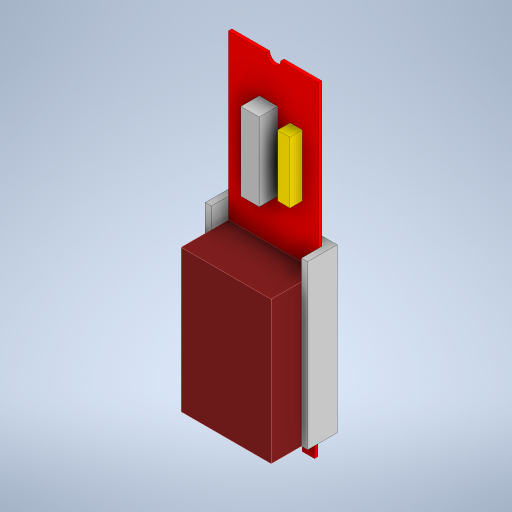
# Autodesk Inventor part: EGPL-T101-C1
Saved by Autodesk Inventor 2024.2 (Build 282272000, 272)
## iProperties
Created: 2024-02-23
Part Number: EGPL-T101-C1
Material: Generic
Document SubType Name: Modeling
Designer: lgnds
Density: 1 g/cm^3
Appearance: Default
Author: lgnds
Autodesk Inventor part; units mm, degrees
ref_plane "YZ Plane" through (0, 0, 0) normal (1, 0, 0) x (0, 1, 0)
ref_plane "XZ Plane" through (0, 0, 0) normal (0, 1, 0) x (-1, 0, 0)
ref_plane "XY Plane" through (0, 0, 0) normal (0, 0, 1) x (1, 0, 0)
sketch "Sketch1" plane through (0, 0, 0) normal (0, 0, 1) x (1, 0, 0)
  line L0 (-11, -40) -> (11, -40)
  line L1 (11, -40) -> (11, 40)
  line L2 (11, 40) -> (-11, 40)
  line L3 (-11, 40) -> (-11, -40)
  line L4 (-11, -40) -> (11, 40) construction
  line L5 (11, -40) -> (-11, 40) construction
  point P0 (0, 0)
  dimension "d0" = 22
  dimension "d1" = 80
  constraints: 12 end point, 2 midpoint, 2 parallel, 1 horizontal, 1 perpendicular
  measures "d0" distance of L1.end L2.end
  measures "d1" distance of L2.end L0.start
extrude "Extrusion1" add sketch "Sketch1" along normal blind 0.8
sketch "Sketch2" plane through (0, 0, 0.8) normal (0, 0, 1) x (1, 0, 0)
  line L0 (11, -40) -> (11, 40) projected
  line L1 (11, 40) -> (-11, 40) projected
  line L2 (-11, 40) -> (-11, -40) projected
  line L3 (-11, -40) -> (11, -40) projected
  line L4 (-10, -40) -> (-10, -36)
  line L5 (-10, -36) -> (-11, -36)
  line L6 (10, -40) -> (10, -36)
  line L7 (10, -36) -> (11, -36)
  line L8 (-7, -40) -> (-5, -40)
  line L9 (-5, -40) -> (-5, -36)
  line L10 (-5, -36) -> (-7, -36)
  line L11 (-7, -36) -> (-7, -40)
  line L12 (0, 56) -> (0, -56) construction
  line L13 (11, -40) -> (-11, -40)
  line L14 (7, -40) -> (5, -40)
  line L15 (5, -40) -> (5, -36)
  line L16 (5, -36) -> (7, -36)
  line L17 (7, -36) -> (7, -40)
  point P0 (0, 0)
  dimension "d4" = 1
  dimension "d5" = 1
  dimension "d6" = 4
  dimension "d7" = 2
  dimension "d8" = 3
  constraints: 26 end point, 9 point on line, 6 symmetric about line, 3 perpendicular, 2 parallel, 1 horizontal, 1 vertical
  measures "d4" distance between parallel lines of L2 L4
  measures "d5" distance between parallel lines of L0 L6
  measures "d6" distance between parallel lines of L3 L5
  measures "d7" distance between parallel lines of L11 L9
  measures "d8" distance between parallel lines of L4 L11
extrude "Extrusion2" cut sketch "Sketch2" against normal blind 0.8 contours L3 L6 L7 L0 | L3 L15 L16 L17 | L5 L4 L3 L2 | L3 L11 L10 L9
fillet "Fillet1" radius 1 5 edges at (-7, -36, 0.4) (-5, -36, 0.4) (5, -36, 0.4) (7, -36, 0.4) (10, -36, 0.4)
sketch "Sketch3" plane through (0, 0, 0.8) normal (0, 0, 1) x (1, 0, 0)
  line L0 (7, -37) -> (7, -40) projected
  line L1 (7, -40) -> (10, -40) projected
  line L2 (10, -40) -> (10, -37) projected
  arc A0 (11, -36) -> (10, -37) centre (11, -37) ccw projected
  line L3 (11, -36) -> (11, 40) projected
  line L4 (11, 40) -> (-11, 40) projected
  line L5 (-11, 40) -> (-11, -36) projected
  line L6 (-11, -36) -> (-10, -36) projected
  line L7 (-10, -36) -> (-10, -40) projected
  line L8 (-10, -40) -> (-7, -40) projected
  line L9 (-7, -40) -> (-7, -37) projected
  arc A1 (-5, -37) -> (-7, -37) centre (-6, -37) ccw projected
  line L10 (-5, -37) -> (-5, -40) projected
  line L11 (-5, -40) -> (5, -40) projected
  line L12 (5, -40) -> (5, -37) projected
  arc A2 (7, -37) -> (5, -37) centre (6, -37) ccw projected
  line L13 (11, -36) -> (11, 40) projected
  line L14 (-11, 0) -> (11, 0)
  line L15 (11, 0) -> (11, -34.8)
  line L16 (11, -34.8) -> (-11, -34.8)
  line L17 (-11, -34.8) -> (-11, 0)
  point P0 (0, 0)
  point P1 (11, 0)
  dimension "d12" = 5.2
  dimension "d13" = 40
  constraints: 8 end point, 2 parallel, 2 point on line, 1 horizontal, 1 perpendicular
  measures "d12" distance between parallel lines of L11 L16
  measures "d13" distance between parallel lines of L11 L14
extrude "Extrusion3" add sketch "Sketch3" along normal blind 11.6 separate body contours L16 L5 L14 L3
sketch "Sketch4" plane through (0, 0, 0) normal (0, 0, -1) x (-1, 0, 0)
  line L0 (-12.5, -34.8) -> (12.5, -34.8)
  line L1 (12.5, -34.8) -> (12.5, 5)
  line L2 (12.5, 5) -> (-12.5, 5)
  line L3 (-12.5, 5) -> (-12.5, -34.8)
  line L4 (11, -34.8) -> (-11, -34.8) projected
  line L5 (-11, -36) -> (-11, 40) projected
  line L6 (11, 40) -> (11, -36) projected
  line L7 (-7, -40) -> (-10, -40) projected
  point P0 (0, 0)
  point P1 (0, -34.8)
  point P2 (-8.5, -40)
  point P3 (11, 5)
  point P4 (-11, 5)
  dimension "d16" = 1.5
  dimension "d17" = 1.5
  dimension "d18" = 45
  constraints: 8 end point, 3 midpoint, 2 parallel, 1 horizontal, 1 perpendicular
  measures "d16" distance between parallel lines of L5 L3
  measures "d17" distance between parallel lines of L6 L1
  measures "d18" distance from line of point (-8.5, -40) L2
extrude "Extrusion4" add sketch "Sketch4" along normal blind 2.2 separate body
sketch "Sketch5" plane through (0, 0, 0) normal (0, 0, 1) x (1, 0, 0)
  line L0 (-12.5, 5) -> (12.5, 5) projected
  line L1 (-12.5, -34.8) -> (-12.5, 5) projected
  line L2 (12.5, -34.8) -> (-12.5, -34.8) projected
  line L3 (12.5, 5) -> (12.5, -34.8) projected
  line L4 (-11, 40) -> (-11, -36) projected
  line L5 (11, -36) -> (11, 40) projected
  point P0 (0, 0)
  point P1 (11, 5)
  point P2 (11, -34.8)
  point P3 (-11, -34.8)
  point P4 (-11, 5)
extrude "Extrusion5" add sketch "Sketch5" along normal blind 5 contours L0 L4 L2 L1 | L0 L3 L2 L5 bodies 3
sketch "Sketch6" plane through (0, 0, 0) normal (0, 0, -1) x (-1, 0, 0)
  line L0 (-11, 40) -> (11, 40) projected
  circle A0 centre (0, 40) radius 1.75
  point P0 (0, 0)
  point P1 (1.75, 40)
  point P2 (-1.75, 40)
  dimension "d23" = 3.5
  constraints: 1 centre point, 1 midpoint
  measures "d23" diameter of A0
extrude "Extrusion6" cut sketch "Sketch6" against normal blind 12.4 contours L0 A0 picked at (-0.4366, 39.6132) bodies 1
sketch "Sketch7" plane through (0, 0, 0.8) normal (0, 0, 1) x (1, 0, 0)
  line L0 (4, 13) -> (7, 13)
  line L1 (7, 13) -> (7, 28)
  line L2 (7, 28) -> (4, 28)
  line L3 (4, 28) -> (4, 13)
  line L4 (4, 13) -> (7, 28) construction
  line L5 (7, 13) -> (4, 28) construction
  line L6 (11, 40) -> (1.75, 40) projected
  line L7 (11, -36) -> (11, 40) projected
  point P0 (0, 0)
  point P1 (5.5, 20.5)
  point P2 (6.375, 40)
  dimension "d26" = 3
  dimension "d27" = 15
  dimension "d28" = 12
  dimension "d29" = 4
  constraints: 12 end point, 3 midpoint, 2 parallel, 1 horizontal, 1 perpendicular
  measures "d26" distance between parallel lines of L1 L3
  measures "d27" distance between parallel lines of L0 L2
  measures "d28" distance from line of point (6.375, 40) L2
  measures "d29" distance between parallel lines of L7 L1
extrude "Extrusion7" add sketch "Sketch7" along normal blind 3 separate body
sketch "Sketch8" plane through (0, 0, 0.8) normal (0, 0, 1) x (1, 0, 0)
  line L0 (-3.5, 30) -> (1, 30)
  line L1 (1, 30) -> (1, 11)
  line L2 (1, 11) -> (-3.5, 11)
  line L3 (-3.5, 11) -> (-3.5, 30)
  line L4 (-1.75, 40) -> (-11, 40) projected
  line L5 (4, 13) -> (7, 13) projected
  line L6 (7, 28) -> (4, 28) projected
  line L7 (4, 28) -> (4, 13) projected
  point P0 (0, 0)
  point P1 (-1.25, 30)
  dimension "d32" = 4.5
  dimension "d34" = 2
  dimension "d35" = 2
  dimension "d36" = 3
  constraints: 8 end point, 2 parallel, 1 horizontal, 1 midpoint, 1 perpendicular
  measures "d32" distance between parallel lines of L1 L3
  measures "d34" distance between parallel lines of L5 L2
  measures "d35" distance from line of point (-1.25, 30) L6
  measures "d36" distance between parallel lines of L7 L1
extrude "Extrusion8" add sketch "Sketch8" along normal blind 4.5 separate body
equation "\"d5\" = d4"
equation "\"d17\" = d16"
equation "\"d34\" = d35"
body "Solid1"
body "Solid2"
body "Solid3"
body "Solid5"
body "Solid6"
